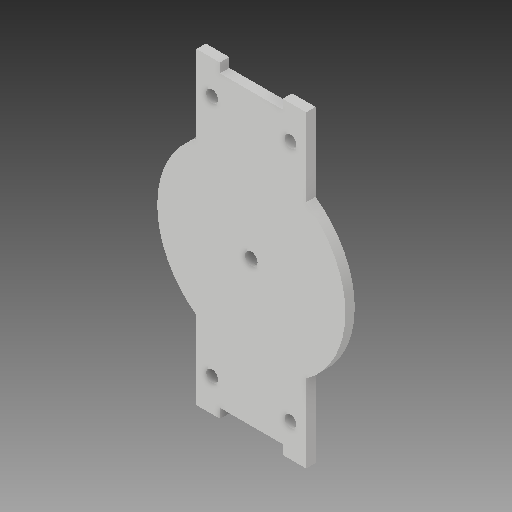
# Autodesk Inventor part: Camera raiser
Saved by Autodesk Inventor 2018 (Build 220112000, 112)
## iProperties
Created: 2018-06-25
Part Number: Camera raiser
Material: Generic
Document SubType Name: Modeling
Designer: Ajith Thomas
Density: 1 g/cm^3
Appearance: Default
Author: Ajith Thomas
Autodesk Inventor part; units mm, degrees
ref_plane "YZ Plane" through (0, 0, 0) normal (1, 0, 0) x (0, 1, 0)
ref_plane "XZ Plane" through (0, 0, 0) normal (0, 1, 0) x (-1, 0, 0)
ref_plane "XY Plane" through (0, 0, 0) normal (0, 0, 1) x (1, 0, 0)
sketch "Sketch1" plane through (0, 0, 0) normal (0, 0, 1) x (1, 0, 0)
  line L0 (0, 0) -> (20, 0) projected
  line L1 (20, 0) -> (20, 3) projected
  line L2 (0, 3) -> (20, 3) projected
  line L3 (0, 0) -> (0, 3) projected
  line L4 (0, -95.4) -> (20, -95.4) projected
  line L5 (20, -95.4) -> (20, -92.4) projected
  line L6 (0, -92.4) -> (20, -92.4) projected
  line L7 (0, -95.4) -> (0, -92.4) projected
  line L8 (-7.5, 3) -> (0, 3) construction
  line L9 (20, 3) -> (27.5, 3) construction
  line L10 (20, -95.4) -> (27.5, -95.4) construction
  line L11 (-7.5, -95.4) -> (0, -95.4) construction
  line L12 (-7.5, 3) -> (27.5, 3)
  line L13 (27.5, -95.4) -> (-7.5, -95.4)
  line L14 (-7.5, 3) -> (27.5, -95.4) construction
  line L15 (27.5, 3) -> (-7.5, -95.4) construction
  line L16 (-7.5, -95.4) -> (-7.5, -70.567)
  line L17 (-7.5, -21.833) -> (-7.5, 3)
  line L18 (27.5, 3) -> (27.5, -21.833)
  line L19 (27.5, -70.567) -> (27.5, -95.4)
  arc A0 (27.5, -70.567) -> (27.5, -21.833) centre (10, -46.2) ccw
  arc A1 (-7.5, -21.833) -> (-7.5, -70.567) centre (10, -46.2) ccw
  dimension "d1" = 35
  dimension "d2" = 35
  constraints: 16 end point, 5 parallel, 4 point on circle, 2 centre point, 2 perpendicular, 1 horizontal, 1 midpoint
  measures "d1" distance between parallel lines of L18 L17
  measures "d2" distance between parallel lines of L19 L16
extrude "Extrusion1" add sketch "Sketch1" against normal blind 3 contours L0 L1 L12 L18 A0 L19 L13 L5 L6 L7 L16 A1 L17 L3
sketch "Sketch2" plane through (0, 0, -3) normal (0, 0, -1) x (-1, 0, 0)
  arc A0 (0.6, -86.2) -> (4.4, -86.2) centre (2.5, -86.2) ccw construction
  line L0 (0.6, -86.2) -> (0.6, -83.5) construction
  arc A1 (4.4, -83.5) -> (0.6, -83.5) centre (2.5, -83.5) ccw construction
  line L1 (4.4, -83.5) -> (4.4, -86.2) construction
  arc A2 (-1.5, -77.8) -> (-2.5, -78.8) centre (-1.5, -78.8) ccw construction
  line L2 (-2.5, -78.8) -> (-2.5, -91.4) construction
  line L3 (-2.5, -91.4) -> (7.5, -91.4) construction
  line L4 (7.5, -91.4) -> (7.5, -78.8) construction
  arc A3 (7.5, -78.8) -> (6.5, -77.8) centre (6.5, -78.8) ccw construction
  line L5 (6.5, -77.8) -> (-1.5, -77.8) construction
  arc A4 (-24.4, -86.2) -> (-20.6, -86.2) centre (-22.5, -86.2) ccw construction
  line L6 (-24.4, -86.2) -> (-24.4, -83.5) construction
  arc A5 (-20.6, -83.5) -> (-24.4, -83.5) centre (-22.5, -83.5) ccw construction
  line L7 (-20.6, -83.5) -> (-20.6, -86.2) construction
  arc A6 (-26.5, -77.8) -> (-27.5, -78.8) centre (-26.5, -78.8) ccw construction
  line L8 (-27.5, -78.8) -> (-27.5, -91.4) construction
  line L9 (-27.5, -91.4) -> (-17.5, -91.4) construction
  line L10 (-17.5, -91.4) -> (-17.5, -78.8) construction
  arc A7 (-17.5, -78.8) -> (-18.5, -77.8) centre (-18.5, -78.8) ccw construction
  line L11 (-18.5, -77.8) -> (-26.5, -77.8) construction
  arc A8 (4.4, -6.2) -> (0.6, -6.2) centre (2.5, -6.2) ccw construction
  line L12 (4.4, -6.2) -> (4.4, -8.9) construction
  arc A9 (0.6, -8.9) -> (4.4, -8.9) centre (2.5, -8.9) ccw construction
  line L13 (0.6, -8.9) -> (0.6, -6.2) construction
  arc A10 (6.5, -14.6) -> (7.5, -13.6) centre (6.5, -13.6) ccw construction
  line L14 (7.5, -13.6) -> (7.5, -1) construction
  line L15 (7.5, -1) -> (-2.5, -1) construction
  line L16 (-2.5, -1) -> (-2.5, -13.6) construction
  arc A11 (-2.5, -13.6) -> (-1.5, -14.6) centre (-1.5, -13.6) ccw construction
  line L17 (-1.5, -14.6) -> (6.5, -14.6) construction
  arc A12 (-20.6, -6.2) -> (-24.4, -6.2) centre (-22.5, -6.2) ccw construction
  line L18 (-20.6, -6.2) -> (-20.6, -8.9) construction
  arc A13 (-24.4, -8.9) -> (-20.6, -8.9) centre (-22.5, -8.9) ccw construction
  line L19 (-24.4, -8.9) -> (-24.4, -6.2) construction
  arc A14 (-18.5, -14.6) -> (-17.5, -13.6) centre (-18.5, -13.6) ccw construction
  line L20 (-17.5, -13.6) -> (-17.5, -1) construction
  line L21 (-17.5, -1) -> (-27.5, -1) construction
  line L22 (-27.5, -1) -> (-27.5, -13.6) construction
  arc A15 (-27.5, -13.6) -> (-26.5, -14.6) centre (-26.5, -13.6) ccw construction
  line L23 (-26.5, -14.6) -> (-18.5, -14.6) construction
  line L24 (-22.5, -86.2) -> (-22.5, -83.5) construction
  line L25 (2.5, -86.2) -> (2.5, -83.5) construction
  line L26 (2.5, -8.9) -> (2.5, -6.2) construction
  line L27 (-22.5, -8.9) -> (-22.5, -6.2) construction
  circle A16 centre (-22.5, -84.85) radius 1.9
  circle A17 centre (2.5, -84.85) radius 1.9
  circle A18 centre (2.5, -7.55) radius 1.9
  circle A19 centre (-22.5, -7.55) radius 1.9
  point P0 (0, 0)
  constraints: 8 end point, 4 centre point, 4 midpoint, 4 vertical
extrude "Extrusion2" cut sketch "Sketch2" against normal blind 27.1625
sketch "Sketch3" plane through (0, 0, 0) normal (0, 0, 1) x (1, 0, 0)
  arc A0 (27.5, -70.567) -> (27.5, -21.833) centre (10, -46.2) ccw projected
  arc A1 (-7.5, -21.833) -> (-7.5, -70.567) centre (10, -46.2) ccw projected
  circle A2 centre (10, -46.2) radius 2
  point P0 (0, 0)
  dimension "d7" = 4
  constraints: 1 centre point, 1 coincident
  measures "d7" diameter of A2
extrude "Extrusion3" cut sketch "Sketch3" against normal blind 14.4625
body "Solid1"
